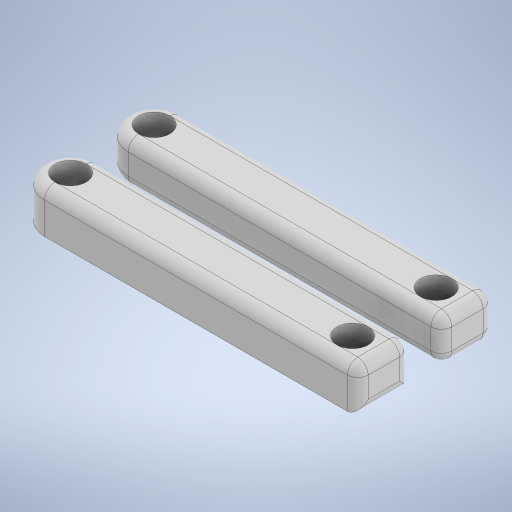
# Autodesk Inventor part: lacznik
Saved by Autodesk Inventor 2024.1 (Build 281209000, 209)
## iProperties
Created: 2023-11-11
Part Number: lacznik
Material: Generic
Document SubType Name: Modeling
Designer: Igor Sarnowski
Density: 1 g/cm^3
Appearance: Default
Author: Igor Sarnowski
Autodesk Inventor part; units mm, degrees
ref_plane "YZ Plane" through (0, 0, 0) normal (1, 0, 0) x (0, 1, 0)
ref_plane "XZ Plane" through (0, 0, 0) normal (0, 1, 0) x (-1, 0, 0)
ref_plane "XY Plane" through (0, 0, 0) normal (0, 0, 1) x (1, 0, 0)
sketch "Sketch2" plane through (0, 0, 0) normal (0, 1, 0) x (-1, 0, 0)
  circle A0 centre (-41, -29) radius 1.5
  circle A1 centre (-41, -21) radius 1.5
  circle A2 centre (-41, -29) radius 2.5
  circle A3 centre (-41, -21) radius 2.5
  line L0 (-41, -31.5) -> (-71, -31.5)
  line L1 (-71, -31.5) -> (-71, -26.5)
  line L2 (-71, -26.5) -> (-41, -26.5)
  line L3 (-41, -23.5) -> (-71, -23.5)
  line L4 (-71, -23.5) -> (-71, -18.5)
  line L5 (-71, -18.5) -> (-41, -18.5)
  circle A4 centre (-68, -21) radius 1.5
  line L6 (-99.5974, -23.735) -> (-99.5974, -19.9897)
  line L7 (-99.3039, -26.0546) -> (-99.3039, -29.7999)
  circle A5 centre (-68, -29) radius 1.5
  dimension "d40" = 3
  dimension "d41" = 3
  dimension "d47" = 5
  dimension "d48" = 5
  dimension "d49" = 30
  dimension "d58" = 3
  constraints: 16 end point, 6 centre point, 4 point on circle, 3 tangent, 2 coincident, 2 perpendicular, 2 point on line, 1 parallel
  measures "d40" diameter of A1
  measures "d41" diameter of A0
  measures "d47" diameter of A2
  measures "d48" diameter of A3
  measures "d49" distance of L0.start L0.end
  measures "d58" diameter of A5
extrude "Extrusion1" add sketch "Sketch2" along normal blind 4
fillet "Fillet1" radius 1 17 edges at (71, 4, -21) (71, 2, -23.5) (38.5, 4, -21) (56, 4, -18.5) (56, 4, -23.5) (71, 0, -21) (71, 2, -18.5) (38.5, 4, -29) (56, 4, -26.5) (56, 4, -31.5) (71, 4, -29) (71, 0, -29) (38.5, 0, -29) (56, 0, -26.5) (56, 0, -31.5) (71, 2, -26.5) (71, 2, -31.5)
body "Solid1"
